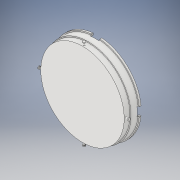
# Autodesk Inventor part: light
Saved by Autodesk Inventor 2019 (Build 230136000, 136)
## iProperties
Created: 2018-07-11
Part Number: light
Material: Generic
Document SubType Name: Modeling
Designer: User
Density: 1 g/cm^3
Appearance: White
Author: User
Autodesk Inventor part; units mm, degrees
ref_plane "YZ Plane" through (0, 0, 0) normal (1, 0, 0) x (0, 1, 0)
ref_plane "XY Plane" through (0, 0, 0) normal (0, 0, 1) x (1, 0, 0)
sketch "Sketch2" plane through (0, 0, 0) normal (1, 0, 0) x (0, 1, 0)
  line L0 (128.4, 0) -> (128.4, 5.5)
  line L1 (128.4, 5.5) -> (125.4, 5.5)
  line L2 (125.4, 5.5) -> (125.4, 27)
  line L3 (125.4, 27) -> (122.4, 27)
  line L4 (122.4, 27) -> (122.4, 44)
  line L5 (122.4, 44) -> (0, 44)
  line L6 (0, 44) -> (0, 41)
  line L7 (0, 41) -> (119.4, 41)
  line L8 (119.4, 41) -> (119.4, 24)
  line L9 (119.4, 24) -> (122.4, 24)
  line L10 (122.4, 24) -> (122.4, 0)
  line L11 (122.4, 0) -> (128.4, 0)
  line L12 (0, 0) -> (0, 41) construction
  line L13 (122.4, 0) -> (0, 0) construction
  line L14 (122.4, 24) -> (122.4, 27) construction
  dimension "d3" = 17
  dimension "d4" = 44
  dimension "d5" = 5.5
  dimension "d6" = 3
  dimension "d8" = 122.4
  constraints: 30 end point, 9 perpendicular, 4 equal length, 2 horizontal, 2 point on line, 2 vertical, 1 coincident
  measures "d3" distance of L3.end L4.end
  measures "d4" distance between parallel lines of L11 L5
  measures "d5" distance of L0.start L0.end
  measures "d6" distance of L2.end L3.end
  measures "d8" distance of L4.end L5.end
revolve "Revolution1" add sketch "Sketch2" angle 360 about axis through (0, 0, 0) along (0, 0, 1)
ref_plane "Work Plane1" through (0, 122.4, 35.5) normal (0, 1, 0) x (-1, 0, 0)
sketch "Sketch4" plane through (0, 122.4, 35.5) normal (0, 1, 0) x (-1, 0, 0)
  circle A0 centre (0, 3.7717) radius 2.25
  line L0 (-122.4, 8.5) -> (122.4, 8.5) projected
  line L1 (0, 3.7717) -> (0, 8.5) construction
  point P0 (0, -35.5)
  dimension "d9" = 4.5
  constraints: 2 end point, 1 centre point, 1 midpoint, 1 perpendicular
  measures "d9" diameter of A0
extrude "Extrusion2" add sketch "Sketch4" along normal blind 7.62
sketch "Sketch5" plane through (0, 130.02, 39.2717) normal (0, 1, 0) x (1, 0, 0)
  arc A0 (0, 2.25) -> (0, -2.25) centre (0, 0) ccw projected
  circle A1 centre (0, 0) radius 3.9236
  point P0 (0, 39.2717)
  constraints: 1 centre point, 1 coincident
extrude "Extrusion3" add sketch "Sketch5" along normal blind 2.54
pattern_circular "Circular Pattern1" count 4 over 360 about axis through (0, 0, 35.5) along (0, 0, -1) of "Extrusion2", "Extrusion3"
sketch "Sketch6" plane through (0, 122.4, 35.5) normal (0, 1, 0) x (-1, 0, 0)
  line L0 (-128.4, -35.5) -> (128.4, -35.5) projected
  line L1 (-122.4, -35.5) -> (122.4, -35.5) projected
  line L2 (12.7, -26.5844) -> (-12.7, -26.5844)
  line L3 (-12.7, -26.5844) -> (-12.7, -35.5)
  line L4 (-12.7, -35.5) -> (12.7, -35.5)
  line L5 (12.7, -35.5) -> (12.7, -26.5844)
  line L6 (12.7, -26.5844) -> (-12.7, -35.5) construction
  line L7 (-12.7, -26.5844) -> (12.7, -35.5) construction
  line L8 (0, -31.0422) -> (0, -35.5) construction
  dimension "d20" = 25.4
  constraints: 14 end point, 2 midpoint, 2 parallel, 2 perpendicular, 1 horizontal, 1 point on line
  measures "d20" distance of L2.start L2.end
extrude "Extrusion4" cut sketch "Sketch6" along normal mid plane 25.4
pattern_circular "Circular Pattern2" count 4 over 360 about axis through (0, 0, 35.5) along (0, 0, -1) of "Extrusion4"
body "Solid2"
